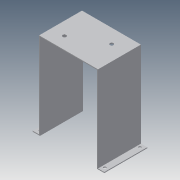
# Autodesk Inventor part: breaker mount
Saved by Autodesk Inventor 2014 (Build 180170000, 170)
## iProperties
Created: 2016-01-13
Part Number: breaker mount
Material: Generic
Document SubType Name: Modeling
Designer: Paul
Density: 1 g/cm^3
Appearance: Default
Author: Paul
Autodesk Inventor part; units mm, degrees
ref_plane "YZ Plane" through (0, 0, 0) normal (1, 0, 0) x (0, 1, 0)
ref_plane "XZ Plane" through (0, 0, 0) normal (0, 1, 0) x (-1, 0, 0)
ref_plane "XY Plane" through (0, 0, 0) normal (0, 0, 1) x (1, 0, 0)
sketch "Sketch1" plane through (0, 0, 0) normal (0, 0, 1) x (1, 0, 0)
  line L0 (-12.7, 0) -> (0, 0)
  line L1 (0, 0) -> (0, 152.4)
  line L2 (0, 152.4) -> (101.6, 152.4)
  line L3 (101.6, 152.4) -> (101.6, 0)
  line L4 (101.6, 0) -> (114.3, 0)
  line L5 (114.3, 1.524) -> (103.124, 1.524)
  line L6 (103.124, 1.524) -> (103.124, 153.924)
  line L7 (103.124, 153.924) -> (-1.524, 153.924)
  line L8 (-1.524, 153.924) -> (-1.524, 1.524)
  line L9 (-1.524, 1.524) -> (-12.7, 1.524)
  line L10 (-12.7, 1.524) -> (-12.7, 0)
  line L11 (114.3, 1.524) -> (114.3, 0)
  dimension "d0" = 152.4
  dimension "d1" = 101.6
  dimension "d3" = 12.7
  dimension "d4" = 12.7
  dimension "d5" = 1.524
  constraints: 24 end point, 5 parallel, 4 collinear, 3 perpendicular, 1 horizontal, 4 other
  measures "d0" distance of L0.end L1.end
  measures "d1" distance of L1.end L2.end
  measures "d3" distance of L3.end L4.end
  measures "d4" distance of L0.start L0.end
  measures "d5" distance between parallel lines of L9 L0
extrude "Extrusion1" add sketch "Sketch1" along normal blind 76.2
sketch "Sketch2" plane through (101.6, 0, 0) normal (0, -1, 0) x (1, 0, 0)
  line L0 (-101.6, 0) -> (-114.3, 0) projected
  line L1 (-101.6, 0) -> (-101.6, 76.2) projected
  line L2 (-114.3, 76.2) -> (-101.6, 76.2) projected
  line L3 (-114.3, 0) -> (-114.3, 76.2) projected
  point P0 (-107.95, 68.9797)
  point P1 (-107.95, 6.4717)
  point P2 (6.35, 68.9797)
  point P3 (6.35, 6.4717)
hole "Hole1" at (-6.35, 0, 68.9797) at (-6.35, 0, 6.4717) at (107.95, 0, 68.9797) at (107.95, 0, 6.4717) direction (0, 1, 0) diameter 4.826 depth 25.4 tip angle 118
sketch "Sketch3" plane through (-1.524, 153.924, 0) normal (0, 1, 0) x (1, 0, 0)
  line L0 (18.6116, -64.0053) -> (82.7466, -64.0053)
  line L1 (87.5091, -59.2428) -> (87.5091, -20.5078)
  line L2 (82.7466, -15.7453) -> (18.6116, -15.7453)
  line L3 (13.8491, -20.5078) -> (13.8491, -59.2428)
  arc A0 (13.8491, -59.2428) -> (18.6116, -64.0053) centre (18.6116, -59.2428) ccw
  arc A1 (18.6116, -15.7453) -> (13.8491, -20.5078) centre (18.6116, -20.5078) ccw
  arc A2 (87.5091, -20.5078) -> (82.7466, -15.7453) centre (82.7466, -20.5078) ccw
  arc A3 (82.7466, -64.0053) -> (87.5091, -59.2428) centre (82.7466, -59.2428) ccw
  circle A4 centre (23.3741, -54.4803) radius 3.175
  circle A5 centre (77.9841, -25.2703) radius 3.175
  point P0 (1.524, 0)
  point P1 (13.8491, -64.0053)
  point P2 (87.5091, -15.7453)
  point P3 (87.5091, -64.0053)
  point P4 (13.8491, -15.7453)
  dimension "d15" = 73.66
  dimension "d16" = 48.26
  dimension "d17" = 4.7625
  dimension "d18" = 6.35
  dimension "d19" = 6.35
  dimension "d20" = 9.525
  dimension "d21" = 9.525
  dimension "d22" = 9.525
  dimension "d23" = 9.525
  constraints: 8 end point, 8 point on circle, 8 point on line, 8 tangent, 6 centre point, 3 equal radius, 2 parallel, 1 horizontal, 1 perpendicular
  measures "d15" distance of point (13.849, -15.745) point (87.509, -15.745)
  measures "d16" distance of point (87.509, -15.745) point (87.509, -64.005)
  measures "d17" radius of A0
  measures "d18" diameter of A4
  measures "d19" diameter of A5
  measures "d20" distance from line of A4.centre L3
  measures "d21" distance from line of A4.centre L0
  measures "d22" distance from line of L1 A5.centre
  measures "d23" distance from line of A5.centre L2
extrude "Extrusion2" cut sketch "Sketch3" against normal blind 76.2 contours A4 | A5
body "Solid1"
